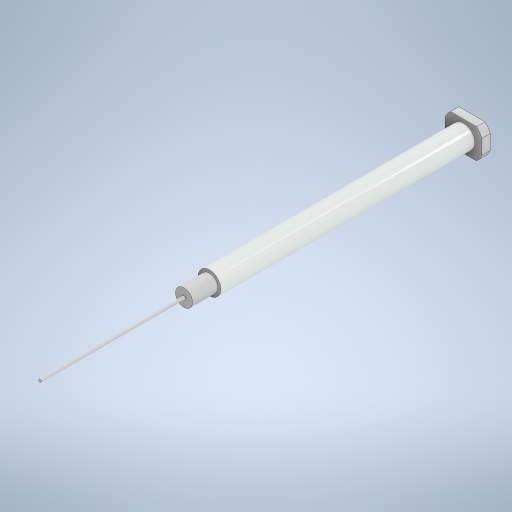
# Autodesk Inventor part: hamilton 100micl syringe body (no plunger)
Saved by Autodesk Inventor 2023.2 (Build 272271000, 271)
## iProperties
Created: 2023-03-16
Part Number: hamilton 100micl syringe body (no plunger)
Material: Generic
Document SubType Name: Modeling
Designer: dmargari
Density: 1 g/cm^3
Appearance: Default
Author: dmargari
Autodesk Inventor part; units mm, degrees
ref_plane "YZ Plane" through (0, 0, 0) normal (1, 0, 0) x (0, 1, 0)
ref_plane "XZ Plane" through (0, 0, 0) normal (0, 1, 0) x (-1, 0, 0)
ref_plane "XY Plane" through (0, 0, 0) normal (0, 0, 1) x (1, 0, 0)
sketch "Sketch1" plane through (0, 0, 0) normal (0, 0, 1) x (1, 0, 0)
  circle A0 centre (26.2216, 22.6561) radius 4
  point P0 (0, 0)
  dimension "d0" = 8
  constraints: 1 centre point
  measures "d0" diameter of A0
extrude "Extrusion1" add sketch "Sketch1" along normal blind 99
sketch "Sketch2" plane through (26.2216, 22.6561, 99) normal (0, 0, 1) x (1, 0, 0)
  circle A0 centre (0, 0) radius 4 projected
  circle A1 centre (0, 0) radius 3
  point P0 (-26.2216, -22.6561)
  dimension "d3" = 6
  constraints: 1 centre point, 1 coincident
  measures "d3" diameter of A1
extrude "Extrusion2" cut sketch "Sketch2" against normal blind 9
sketch "Sketch3" plane through (26.2216, 22.6561, 99) normal (0, 0, 1) x (1, 0, 0)
  circle A0 centre (0, 0) radius 0.75
  point P0 (-26.2216, -22.6561)
  dimension "d6" = 1.5
  constraints: 1 centre point
  measures "d6" diameter of A0
extrude "Extrusion3" cut sketch "Sketch3" against normal through all
sketch "Sketch5" plane through (26.2216, 22.6561, 99) normal (0, 0, 1) x (1, 0, 0)
  circle A0 centre (0, 0) radius 0.75 projected
  circle A1 centre (0, 0) radius 0.5
  point P0 (-26.2216, -22.6561)
  dimension "d9" = 1
  constraints: 1 centre point, 1 coincident
  measures "d9" diameter of A1
extrude "Extrusion4" add sketch "Sketch5" along normal blind 51 contours A1
sketch "Sketch6" plane through (26.2216, 22.6561, 0) normal (0, 0, -1) x (-1, 0, 0)
  circle A0 centre (0, 0) radius 4 projected
  line L0 (-6.5, -5.25) -> (6.5, -5.25)
  line L1 (6.5, -5.25) -> (6.5, 5.25)
  line L2 (6.5, 5.25) -> (-6.5, 5.25)
  line L3 (-6.5, 5.25) -> (-6.5, -5.25)
  circle A1 centre (0, 0) radius 0.75 projected
  line L4 (-6.5, -5.25) -> (6.5, 5.25) construction
  line L5 (6.5, -5.25) -> (-6.5, 5.25) construction
  circle A2 centre (0, 0) radius 7
  point P0 (26.2216, -22.6561)
  point P1 (-4.6301, -5.25)
  point P2 (-6.5, -2.5981)
  point P3 (-6.5, 2.5981)
  point P4 (-4.6301, 5.25)
  point P5 (4.6301, 5.25)
  point P6 (6.5, 2.5981)
  point P7 (6.5, -2.5981)
  point P8 (4.6301, -5.25)
  dimension "d12" = 13
  dimension "d13" = 10.5
  dimension "d16" = 14
  constraints: 12 end point, 2 midpoint, 2 parallel, 1 centre point, 1 coincident, 1 horizontal, 1 perpendicular
  measures "d12" distance of L2.end L1.end
  measures "d13" distance of L1.end L0.end
  measures "d16" diameter of A2
extrude "Extrusion5" add sketch "Sketch6" along normal blind 3 contours A0 | L3 A2 L0 | A2 L3 L2 L1 L0 | A2 L1 L0 | L3 L2 A2 | A2 L2 L1
extrude "Extrusion6" cut sketch "Sketch6" along normal blind 3 contours L3 A2 L0 | A2 L1 L0 | L3 L2 A2 | A2 L2 L1
body "Solid1"
